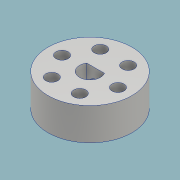
# Autodesk Inventor part: AA055
Saved by Autodesk Inventor 2017 SP1 (Build 210196100, 196)
## iProperties
Created: 2018-06-22
Part Number: AA055
Material: Aluminum 6061
Document SubType Name: Modeling
Designer: Zach
Density: 2.7 g/cm^3
Appearance: Aluminum - Flat
Author: Zach
Autodesk Inventor part; units mm, degrees
ref_plane "YZ Plane" through (0, 0, 0) normal (1, 0, 0) x (0, 1, 0)
ref_plane "XZ Plane" through (0, 0, 0) normal (0, 1, 0) x (-1, 0, 0)
ref_plane "XY Plane" through (0, 0, 0) normal (0, 0, 1) x (1, 0, 0)
sketch "Sketch9" plane through (0, 0, 0) normal (0, 0, 1) x (1, 0, 0)
  circle A0 centre (0, 0) radius 4.125 construction
  circle A1 centre (0, 0) radius 16.5
  circle A2 centre (11, 0) radius 2.4
  circle A3 centre (5.5, 9.5263) radius 2.4
  circle A4 centre (-5.5, 9.5263) radius 2.4
  line L0 (-3.4894, 2.2) -> (3.4894, 2.2)
  arc A5 (-3.4894, 2.2) -> (3.4894, 2.2) centre (0, 0) ccw
  circle A6 centre (-11, 0) radius 2.4
  circle A7 centre (-5.5, -9.5263) radius 2.4
  circle A8 centre (5.5, -9.5263) radius 2.4
  dimension "d25" = 8.25
  dimension "d26" = 33
  dimension "d27" = 4.8
  dimension "d31" = 360
  dimension "d33" = 2.2
  dimension "d36" = 11
  constraints: 9 centre point, 4 point on circle, 3 coincident, 2 concentric, 2 end point, 1 horizontal, 1 horizontal alignment, 13 other
  measures "d25" diameter of A0
  measures "d26" diameter of A1
  measures "d27" diameter of A2
  measures "d33" distance from line of point (0, 0) L0
  measures "d36" distance of point (0, 0) A2.centre
extrude "Extrusion8" add sketch "Sketch9" along normal blind 12.7
sketch "Sketch10" plane through (-3.4894, 2.2, 0) normal (0, -1, 0) x (1, 0, 0)
  line L0 (6.9787, 0) -> (0, 0) projected
  line L1 (6.9787, 0) -> (6.9787, 12.7) projected
  line L2 (0, 12.7) -> (6.9787, 12.7) projected
  line L3 (0, 0) -> (0, 12.7) projected
  circle A0 centre (3.4894, 6.35) radius 2.5
  point P0 (3.4894, 0)
  point P1 (3.4894, 12.7)
  point P2 (0, 6.35)
  dimension "d37" = 5
  constraints: 2 midpoint, 1 centre point, 1 horizontal alignment, 1 vertical alignment
  measures "d37" diameter of A0
extrude "Extrusion9" cut sketch "Sketch10" against normal through all contours A0
body "Solid2"
